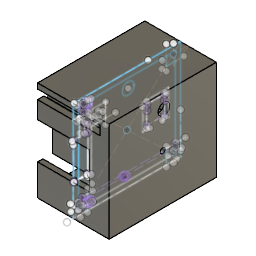
Light and Temp sensor v1 (Autodesk Fusion 360 design; units mm, degrees)
Autodesk Fusion 360 part; units mm, degrees
sketch "DHT22" plane through (0, 0, 0) normal (0, 0, 1) x (1, 0, 0)
  line L0 (7.5, -10) -> (-7.5, -10)
  line L1 (-7.5, -10) -> (-7.5, 10)
  line L2 (-7.5, 10) -> (7.5, 10)
  line L3 (7.5, 10) -> (7.5, -10)
  line L4 (7.5, -10) -> (-7.5, 10) construction
  line L5 (-7.5, -10) -> (7.5, 10) construction
  line L6 (-16.1042, 15) -> (19.3546, 15) construction
  line L7 (7.5, 10) -> (4.6132, 15)
  line L8 (0, -2.0118) -> (0, 2.0118) construction
  line L9 (-3.2444, 0) -> (3.2444, 0) construction
  line L10 (-7.5, 10) -> (-4.6132, 15)
  line L11 (-4.6132, 15) -> (4.6132, 15)
  line L12 (-8.5762, 12.5) -> (8.9313, 12.5) construction
  line L13 (0, 15.9476) -> (0, 9.0438) construction
  circle A0 centre (0, 12.4957) radius 1.4
  line L14 (-5.5335, -10) -> (-5.5335, -18)
  line L15 (-5.0335, -10) -> (-5.0335, -18)
  line L16 (-5.5335, -18) -> (-5.0335, -18)
  line L17 (-1.7002, -10) -> (-1.7002, -18)
  line L18 (-2.2002, -18) -> (-1.7002, -18)
  line L19 (-2.2002, -10) -> (-2.2002, -18)
  line L20 (1.6331, -10) -> (1.6331, -18)
  line L21 (1.1331, -18) -> (1.6331, -18)
  line L22 (1.1331, -10) -> (1.1331, -18)
  line L23 (4.9665, -10) -> (4.9665, -18)
  line L24 (4.4665, -18) -> (4.9665, -18)
  line L25 (4.4665, -10) -> (4.4665, -18)
  dimension "d1" = 15
  dimension "d2" = 20
  dimension "d3" = 15
  dimension "d4" = 60
  dimension "d5" = 2.8
  dimension "d6" = 8
  dimension "d7" = 0.5
  dimension "d10" = 10
  dimension "d11" = 0
  constraint horizontal L0
  constraint perpendicular L0 L1
  constraint parallel L0 L2
  constraint parallel L1 L3
  constraint coincident L4 origin
  constraint coincident L5 origin
  constraint perpendicular L1 L6
  constraint coincident L6 L7.end
  constraint vertical L8
  constraint perpendicular L8 L9
  constraint midpoint origin L8
  constraint midpoint origin L9
  constraint symmetric L2.end L8 L1.end
  constraint symmetric L7.end L8 L10.end
  constraint horizontal L12
  constraint perpendicular L12 L13
  constraint symmetric L2.end L1.end L13
  constraint midpoint L13 A0.centre
  constraint coincident L0 L14.start
  constraint perpendicular L0 L14
  constraint coincident L0 L15.start
  constraint perpendicular L0 L15
  constraint equal L14 L15
  measures "d1" distance of L1.end L2.end
  measures "d2" distance of L0.end L1.end
  measures "d3" distance of origin L6
  measures "d4" angle of L6 L7
  measures "d5" diameter of A0
  measures "d6" distance of L0 L14.end
  measures "d7" distance of L14 L15
extrude "Extrude1" add sketch "DHT22" along normal blind 7.7 contours L0 L1 L2 L3 makes body 1 in component "DHT22"
extrude "Extrude2" add sketch "DHT22" along normal blind 1.5 contours L2 L7 L10 L11 bodies 1 in component "DHT22"
extrude "Extrude3" add sketch "DHT22" along normal blind 4.1 and the other way blind -3.6 contours L0 L23 L24 L25 | L0 L20 L21 L22 | L0 L14 L15 L16 | L0 L17 L18 L19 bodies 1 in component "DHT22"
sketch "Light sensor" plane through (0, 0, 0) normal (0, 0, 1) x (1, 0, 0)
  line L0 (-2.4, 4.9216) -> (-2.4, -4.8279) construction
  line L1 (2.4, 4.9216) -> (2.4, -4.8279) construction
  line L2 (-3.4686, 2.05) -> (2.8124, 2.05) construction
  line L3 (-3.4686, -2.05) -> (1.4, -2.05) construction
  line L4 (0, -1.3974) -> (0, 1.3974) construction
  line L5 (1.6915, 0) -> (-1.6915, 0) construction
  line L6 (-1.4, 2.05) -> (1.4, 2.05)
  line L7 (2.4, 1.05) -> (2.4, -1.05)
  line L8 (2.4, -2.05) -> (-1.4, -2.05)
  line L9 (-2.4, -1.05) -> (-2.4, 1.05)
  arc A0 (-1.4, 2.05) -> (-2.4, 1.05) centre (-1.4, 1.05) ccw
  arc A1 (2.4, 1.05) -> (1.4, 2.05) centre (1.4, 1.05) ccw
  arc A2 (-2.4, -1.05) -> (-1.4, -2.05) centre (-1.4, -1.05) ccw
  arc A3 (1.4, -2.05) -> (2.4, -1.05) centre (1.4, -1.05) ccw
  circle A4 centre (-1.9, 0) radius 0.15
  circle A5 centre (1.9, 0) radius 0.15
  dimension "d20" = 4.8
  dimension "d21" = 4.1
  dimension "d22" = 1
  dimension "d23" = 1
  dimension "d24" = 1
  dimension "d25" = 1
  dimension "d26" = 0.3
  dimension "d27" = 0.5
  constraint vertical L0
  constraint parallel L0 L1
  constraint perpendicular L0 L2
  constraint perpendicular L0 L3
  constraint perpendicular L3 L4
  constraint perpendicular L1 L5
  constraint midpoint origin L5
  constraint midpoint origin L4
  constraint horizontal L6
  constraint vertical L7
  constraint horizontal L8
  constraint vertical L9
  constraint coincident L1 L8.start
  constraint coincident L3 L8.start
  constraint tangent L6 A0
  constraint tangent L9 A0
  constraint tangent L6 A1
  constraint tangent L7 A1
  constraint tangent L8 A2
  constraint tangent L9 A2
  constraint coincident L8.start L7
  constraint tangent L7 A3
  constraint tangent L3 A3
  constraint symmetric L4 A4 A5
  measures "d20" distance of L0 L1
  measures "d21" distance of L2 L3
  measures "d22" radius of A0
  measures "d23" radius of A1
  measures "d24" radius of A2
  measures "d25" radius of A3
  measures "d26" diameter of A4
  measures "d27" distance of L0 A4.centre
extrude "Extrude1'" add sketch "Light sensor" along normal blind 2.3 separate body contours L6 L7 L8 L9 A0 A1 A2 A3 | A4 | A5 makes body 2 in component "Light sensor"
extrude "Extrude2'" add sketch "Light sensor" against normal blind 30 contours A4 | A5 bodies 2 in component "Light sensor"
sketch "ESP32 Wroom-32" plane through (0, 0, 0) normal (0, 0, 1) x (1, 0, 0)
  line L0 (14.1, -44.2458) -> (14.1, 38.8499) construction
  line L1 (-14.1, -44.2458) -> (-14.1, 38.8499) construction
  line L2 (0, -14.9734) -> (0, 14.9734) construction
  line L3 (8.9037, 0) -> (-8.9037, 0) construction
  line L4 (24.487, -25.95) -> (-46.8728, -25.95) construction
  line L5 (24.487, 25.95) -> (-46.8728, 25.95) construction
  line L6 (14.1, -25.95) -> (-14.1, -25.95)
  line L7 (-14.1, -25.95) -> (-14.1, 25.95)
  line L8 (-14.1, 25.95) -> (14.1, 25.95)
  line L9 (14.1, 25.95) -> (14.1, -25.95)
  circle A0 centre (11.3, -23.15) radius 1.6
  circle A1 centre (-11.3, -23.15) radius 1.6
  circle A2 centre (11.3, 23.15) radius 1.6
  circle A3 centre (-11.3, 23.15) radius 1.6
  line L10 (4.4, 20.65) -> (-4.4, 20.65)
  line L11 (-4.4, 20.65) -> (-4.4, 28.05)
  line L12 (-4.4, 28.05) -> (4.4, 28.05)
  line L13 (4.4, 28.05) -> (4.4, 20.65)
  line L14 (8.9, 20.35) -> (6.3, 20.35)
  line L15 (6.3, 20.35) -> (6.3, 24.25)
  line L16 (6.3, 24.25) -> (8.9, 24.25)
  line L17 (8.9, 24.25) -> (8.9, 20.35)
  line L18 (7.6, 22.1367) -> (7.6, 22.6573) construction
  line L19 (8.0941, 22.3) -> (7.6065, 22.3) construction
  circle A4 centre (7.6, 22.3) radius 0.8
  line L20 (15.8445, 24.25) -> (-17.3175, 24.25) construction
  line L21 (-8.9, 24.25) -> (-8.9, 20.35)
  line L22 (-8.9, 20.35) -> (-6.3, 20.35)
  line L23 (-6.3, 20.35) -> (-6.3, 24.25)
  line L24 (-6.3, 24.25) -> (-8.9, 24.25)
  circle A5 centre (-7.6, 22.3) radius 0.8
  line L25 (-3.8, 2.05) -> (-5.8, 2.05)
  line L26 (-5.8, 2.05) -> (-5.8, 3.05)
  line L27 (-5.8, 3.05) -> (-3.8, 3.05)
  line L28 (-3.8, 3.05) -> (-3.8, 2.05)
  line L29 (2.9, 2.05) -> (0.9, 2.05)
  line L30 (0.9, 2.05) -> (0.9, 3.05)
  line L31 (0.9, 3.05) -> (2.9, 3.05)
  line L32 (2.9, 3.05) -> (2.9, 2.05)
  line L33 (13.9, -20.75) -> (11.4, -20.75)
  line L34 (11.4, -20.75) -> (11.4, 17.15)
  line L35 (11.4, 17.15) -> (13.9, 17.15)
  line L36 (13.9, 17.15) -> (13.9, -20.75)
  line L37 (-11.4, -20.75) -> (-11.4, 17.15)
  line L38 (-13.9, -20.75) -> (-11.4, -20.75)
  line L39 (-13.9, 17.15) -> (-13.9, -20.75)
  line L40 (-11.4, 17.15) -> (-13.9, 17.15)
  dimension "d34" = 51.9
  dimension "d35" = 28.2
  dimension "d36" = 3.2
  dimension "d37" = 2.8
  dimension "d38" = 2.8
  dimension "d39" = 8.8
  dimension "d40" = 7.4
  dimension "d41" = 2.1
  dimension "d42" = 2.6
  dimension "d43" = 3.9
  dimension "d44" = 1.6
  dimension "d45" = 1.7
  dimension "d46" = 1.9
  dimension "d47" = 2
  dimension "d48" = 1
  dimension "d49" = 8.3
  dimension "d50" = 22.9
  dimension "d51" = 2
  dimension "d52" = 1
  dimension "d53" = 4.7
  dimension "d54" = 2.5
  dimension "d55" = 37.9
  dimension "d56" = 8.8
  dimension "d57" = 0.2
  constraint vertical L0
  constraint parallel L0 L1
  constraint parallel L1 L2
  constraint perpendicular L2 L4
  constraint perpendicular L0 L5
  constraint symmetric L0 L1 L2
  constraint midpoint origin L2
  constraint midpoint origin L3
  constraint symmetric L3 L4 L5
  constraint horizontal L6
  constraint vertical L7
  constraint horizontal L8
  constraint vertical L9
  constraint coincident L5 L7.end
  constraint coincident L1 L7.end
  constraint coincident L4 L6.start
  constraint coincident L0 L6.start
  constraint symmetric L2 A0 A1
  constraint symmetric L3 A0 A2
  constraint symmetric L3 A1 A3
  constraint horizontal L10
  constraint vertical L11
  constraint horizontal L12
  constraint vertical L13
  constraint symmetric L2 L11 L13
  constraint horizontal L14
  constraint vertical L15
  constraint horizontal L16
  constraint vertical L17
  constraint vertical L18
  constraint perpendicular L18 L19
  constraint symmetric L14 L16 L19
  constraint symmetric L15 L17 L18
  constraint coincident L18 A4.centre
  constraint coincident L19 A4.centre
  constraint perpendicular L9 L20
  constraint collinear L16 L20
  constraint symmetric L2 L14.start L21.end
  constraint symmetric L2 L14.end L22.end
  constraint symmetric L2 L15.end L23.end
  constraint symmetric L2 L16.end L21.start
  constraint symmetric L2 A4 A5
  constraint horizontal L25
  constraint vertical L26
  constraint horizontal L27
  constraint vertical L28
  constraint horizontal L29
  constraint vertical L30
  constraint horizontal L31
  constraint vertical L32
  constraint collinear L27 L31
  constraint horizontal L33
  constraint vertical L34
  constraint horizontal L35
  constraint vertical L36
  constraint symmetric L2 L33.start L38.start
  constraint symmetric L2 L33.end L37.start
  constraint symmetric L2 L34.end L37.end
  constraint symmetric L2 L35.end L39.start
  measures "d34" distance of L4 L5
  measures "d35" distance of L0 L1
  measures "d36" diameter of A0
  measures "d37" distance of L6 A0.centre
  measures "d38" distance of L0 A0.centre
  measures "d39" distance of L10.start L10.end
  measures "d40" distance of L10.start L12.end
  measures "d41" distance of L8 L12
  measures "d42" distance of L14.start L14.end
  measures "d43" distance of L14.start L16.end
  measures "d44" diameter of A4
  measures "d45" distance of L5 L20
  measures "d46" distance of L13 L15
  measures "d47" distance of L25.start L25.end
  measures "d48" distance of L25.start L27.end
  measures "d49" distance of L7 L26
  measures "d50" distance of L8 L27
  measures "d51" distance of L29.start L29.end
  measures "d52" distance of L29.start L31.end
  measures "d53" distance of L28 L30
  measures "d54" distance of L33.start L33.end
  measures "d55" distance of L33.start L35.end
  measures "d56" distance of L8 L35
  measures "d57" distance of L0 L36
extrude "Extrude1''" add sketch "ESP32 Wroom-32" along normal blind 1.5 separate body contours L6 L7 L8 L9 L10 L11 L13 | L8 L10 L11 L13 | L14 L15 L16 L17 | A4 | L21 L22 L23 L24 | A5 | L25 L26 L27 L28 | L29 L30 L31 L32 | L33 L34 L35 L36 | L37 L38 L39 L40 makes body 3 in component "ESP32 Wroom-32"
extrude "Extrude2''" add sketch "ESP32 Wroom-32" along normal blind 4.7 and the other way blind -1.5 contours L8 L10 L11 L13 | L8 L11 L12 L13 bodies 3 in component "ESP32 Wroom-32"
extrude "Extrude3'" add sketch "ESP32 Wroom-32" along normal blind 3.5 and the other way blind -1.5 contours L14 L15 L16 L17 | A4 | L21 L22 L23 L24 | A5 bodies 3 in component "ESP32 Wroom-32"
extrude "Extrude4" add sketch "ESP32 Wroom-32" along normal blind 4.2 and the other way blind -1.5 contours A4 | A5 bodies 3 in component "ESP32 Wroom-32"
extrude "Extrude5" add sketch "ESP32 Wroom-32" along normal blind 2 and the other way blind -1.5 contours L25 L26 L27 L28 | L29 L30 L31 L32 bodies 3 in component "ESP32 Wroom-32"
extrude "Extrude6" add sketch "ESP32 Wroom-32" against normal blind 8.3 contours L33 L34 L35 L36 | L37 L38 L39 L40 bodies 3 in component "ESP32 Wroom-32"
sketch "Screw terminal" plane through (0, 0, 0) normal (0, 0, 1) x (1, 0, 0)
  line L0 (4.9, -4.95) -> (-4.9, -4.95)
  line L1 (-4.9, -4.95) -> (-4.9, 4.95)
  line L2 (-4.9, 4.95) -> (4.9, 4.95)
  line L3 (4.9, 4.95) -> (4.9, -4.95)
  line L4 (0, 1.4194) -> (0, -1.4194) construction
  line L5 (-1.4426, 0) -> (1.4426, 0) construction
  line L6 (4.6, -0.85) -> (0.4, -0.85)
  line L7 (0.4, -0.85) -> (0.4, 4.55)
  line L8 (0.4, 4.55) -> (4.6, 4.55)
  line L9 (4.6, 4.55) -> (4.6, -0.85)
  line L10 (-4.6, 4.55) -> (-4.6, -0.85)
  line L11 (-4.6, -0.85) -> (-0.4, -0.85)
  line L12 (-0.4, -0.85) -> (-0.4, 4.55)
  line L13 (-0.4, 4.55) -> (-4.6, 4.55)
  line L14 (2.65, 4.95) -> (2.35, 4.95)
  line L15 (2.35, 4.95) -> (2.35, 8.45)
  line L16 (2.35, 8.45) -> (2.65, 8.45)
  line L17 (2.65, 8.45) -> (2.65, 4.95)
  line L18 (2.5, 7.4653) -> (2.5, 5.947) construction
  line L19 (-2.35, 4.95) -> (-2.35, 8.45)
  line L20 (-2.65, 4.95) -> (-2.35, 4.95)
  line L21 (-2.65, 8.45) -> (-2.65, 4.95)
  line L22 (-2.35, 8.45) -> (-2.65, 8.45)
  dimension "d78" = 9.8
  dimension "d79" = 9.9
  dimension "d80" = 4.2
  dimension "d81" = 5.4
  dimension "d82" = 4.1
  dimension "d83" = 0.3
  dimension "d84" = 0.3
  dimension "d85" = 3.5
  constraint horizontal L0
  constraint vertical L1
  constraint horizontal L2
  constraint vertical L3
  constraint parallel L1 L4
  constraint perpendicular L4 L5
  constraint midpoint origin L5
  constraint midpoint origin L4
  constraint symmetric L0 L2 L5
  constraint symmetric L1 L3 L4
  constraint horizontal L6
  constraint vertical L7
  constraint horizontal L8
  constraint vertical L9
  constraint symmetric L4 L6.start L10.end
  constraint symmetric L4 L6.end L11.end
  constraint symmetric L4 L7.end L12.end
  constraint symmetric L4 L8.end L10.start
  constraint horizontal L14
  constraint vertical L15
  constraint horizontal L16
  constraint vertical L17
  constraint coincident L2 L14.start
  constraint perpendicular L16 L18
  constraint symmetric L15 L17 L18
  constraint symmetric L7 L9 L18
  constraint symmetric L4 L14.start L20.start
  constraint symmetric L4 L14.end L19.start
  constraint symmetric L4 L15.end L19.end
  constraint symmetric L4 L16.end L21.start
  measures "d78" distance of L0.start L0.end
  measures "d79" distance of L0.start L2.end
  measures "d80" distance of L6.start L6.end
  measures "d81" distance of L6.start L8.end
  measures "d82" distance of L0 L6
  measures "d83" distance of L3 L9
  measures "d84" distance of L14.start L14.end
  measures "d85" distance of L14.start L16.end
extrude "Extrude1'''" add sketch "Screw terminal" along normal blind 7.7 separate body contours L0 L1 L2 L3 L14 L20 | L6 L7 L8 L9 | L10 L11 L12 L13 makes body 4 in component "Screw terminal"
extrude "Extrude2'''" cut sketch "Screw terminal" along normal blind 8 and the other way blind -5 contours L6 L7 L8 L9 | L10 L11 L12 L13 bodies 4 in component "Screw terminal"
extrude "Extrude3''" add sketch "Screw terminal" along normal blind 4.15 and the other way blind -3.85 contours L2 L14 L15 L16 L17 | L2 L19 L20 L21 L22 bodies 4 in component "Screw terminal"
sketch "Sketch1" plane through (0, 0, 0) normal (1, 0, 0) x (0, 1, 0) in component "Screw terminal"
  line L0 (4.95, 0) -> (-4.95, 0)
  line L1 (-4.95, 0) -> (-4.95, 7.7)
  line L2 (-4.95, 7.7) -> (4.95, 7.7)
  line L3 (4.95, 7.7) -> (4.95, 0)
  line L4 (-2.05, 9.7062) -> (-2.05, -0.1924) construction
  line L5 (-6.0619, 6.7) -> (-1.5708, 6.7) construction
  line L6 (-6.0619, 1.7) -> (-1.5708, 1.7) construction
  line L7 (-2.05, 7.7) -> (-4.95, 6.7)
  line L8 (-2.05, 0) -> (-4.95, 1.7)
  line L9 (-2.05, 0) -> (-4.95, 0)
  line L10 (-4.95, 0) -> (-4.95, 1.7)
  line L11 (-4.95, 6.7) -> (-4.95, 7.7)
  line L12 (-4.95, 7.7) -> (-2.05, 7.7)
  dimension "d96" = 7
  dimension "d97" = 5
  dimension "d98" = 1
  constraint perpendicular L0 L4
  constraint perpendicular L4 L5
  constraint perpendicular L4 L6
  constraint coincident L4 L7.start
  constraint coincident L2 L7.start
  constraint coincident L1 L7.end
  constraint coincident L5 L7.end
  constraint coincident L0 L8.start
  constraint coincident L4 L8.start
  constraint coincident L1 L8.end
  constraint coincident L6 L8.end
  constraint coincident L0.end L1.start
  constraint coincident L1.end L2.start
  measures "d96" distance of L3 L4
  measures "d97" distance of L5 L6
  measures "d98" distance of L2 L5
extrude "Extrude4'" cut sketch "Sketch1" along normal mid plane 10 contours L0 L1 L8 L9 L10 | L1 L2 L7 L11 L12 bodies 4 in component "Screw terminal"
sketch "Sketch2" plane through (0, -4.95, 0) normal (0, -1, 0) x (1, 0, 0) in component "Screw terminal"
  line L0 (4.9, 6.7) -> (-4.9, 6.7)
  line L1 (-4.9, 6.7) -> (-4.9, 1.7)
  line L2 (-4.9, 1.7) -> (4.9, 1.7)
  line L3 (4.9, 1.7) -> (4.9, 6.7)
  line L4 (-5.6068, 4.2) -> (5.7003, 4.2) construction
  line L5 (-2.4483, -0.8504) -> (-2.4483, 8.9242) construction
  line L6 (0.0034, -0.7898) -> (0.0034, 0.468) construction
  line L7 (-4.9, 1.7) -> (-4.9, 6.7) construction
  line L8 (4.9, 1.7) -> (4.9, 6.7) construction
  line L9 (-4.9, 1.7) -> (4.9, 1.7) construction
  line L10 (4.9, 6.7) -> (-4.9, 6.7) construction
  circle A0 centre (-2.4483, 4.2) radius 1.75
  circle A1 centre (2.4551, 4.2) radius 1.75
  dimension "d101" = 3.5
  constraint perpendicular L3 L4
  constraint perpendicular L2 L5
  constraint perpendicular L2 L6
  constraint symmetric L0 L4 L9
  constraint coincident L5 A0.centre
  constraint coincident L4 A0.centre
  constraint symmetric L6 A0 A1
  measures "d101" diameter of A0
extrude "Extrude5'" cut sketch "Sketch2" against normal blind 6.5 contours A0 | A1 bodies 4 in component "Screw terminal"
sketch "Box side view" plane through (0, 0, 0) normal (1, 0, 0) x (0, 1, 0)
  line L0 (26.8145, -7.7) -> (-34.5766, -7.7) construction
  line L1 (28.95, -4.6875) -> (28.95, 15.0705) construction
  line L2 (-31.05, -1.5625) -> (-31.05, 27.8729) construction
  line L3 (-20.6653, 4.0827) -> (-20.6653, 36.4415) construction
  line L4 (-27.5, 32.006) -> (-27.5, 37.8528) construction
  line L5 (-30.6451, 48.05) -> (10.7863, 48.05) construction
  line L6 (-28.05, -4.7) -> (-20.65, -4.7) construction
  line L7 (-25.95, -1.5) -> (25.95, -1.5) construction
  line L8 (25.95, 0) -> (-25.95, 0) construction
  line L9 (-30.7, 30) -> (-30.7, 10) construction
  line L10 (-23, 10) -> (-23, 30) construction
  line L11 (-23, 30) -> (-23, 35) construction
  line L12 (-24.5, 35) -> (-24.5, 30) construction
  line L13 (-23, 10) -> (-30.7, 10) construction
  line L14 (10.1, 17.05) -> (10.1, 24.05) construction
  line L15 (19.9, 17.05) -> (10.1, 17.05) construction
  line L16 (19.9, 24.05) -> (19.9, 17.05) construction
  line L17 (25.95, 0) -> (25.95, -1.5) construction
  line L18 (-25.95, 0) -> (-25.95, -1.5) construction
  line L19 (-28.05, -1.5) -> (-28.05, -4.7) construction
  line L20 (-3.05, -2) -> (-2.05, -2) construction
  line L21 (-2.05, -1.5) -> (-2.05, -2) construction
  line L22 (-3.05, -1.5) -> (-3.05, -2) construction
  line L23 (-23.1, -4.2) -> (-21.5, -4.2) construction
  line L24 (-21.5, -3.5) -> (-23.1, -3.5) construction
  line L25 (19.9, 24.05) -> (19.9, 26.95) construction
  line L26 (19.9, 26.95) -> (10.1, 26.95) construction
  line L27 (10.1, 26.95) -> (10.1, 24.05) construction
  line L28 (-23, 35) -> (-24.5, 35) construction
  line L29 (-24.5, 30) -> (-30.7, 30) construction
  line L30 (-23, 40.95) -> (-25.3, 40.95) construction
  line L31 (-23, 41.95) -> (-23, 44.05) construction
  line L32 (-25.3, 44.05) -> (-25.3, 41.95) construction
  line L33 (-23, 45.05) -> (-25.3, 45.05) construction
  line L34 (-31.05, -7.7) -> (-31.05, 48.05)
  line L35 (-31.05, 48.05) -> (28.95, 48.05)
  line L36 (-31.05, -7.7) -> (28.95, -7.7)
  line L37 (28.95, -7.7) -> (28.95, 48.05)
  line L38 (25.95, -4.7) -> (25.95, 45.05)
  line L39 (-28.05, 45.05) -> (25.95, 45.05)
  line L40 (-28.05, -4.7) -> (-28.05, 45.05)
  line L41 (-28.05, -4.7) -> (25.95, -4.7)
  line L42 (-28.9766, 37.95) -> (-22.6639, 37.95) construction
  line L43 (-21, 45.4212) -> (-21, 39.95) construction
  line L44 (-23, 41.95) -> (-23, 40.95) construction
  line L45 (-29.0303, 46.05) -> (-24.1853, 46.05) construction
  line L46 (-27.5, 46.5514) -> (-27.5, 39.1534) construction
  line L47 (-25.3, 35.2) -> (-22.8, 35.2) construction
  line L48 (-24.7, 35.9637) -> (-24.7, 30.5464) construction
  line L49 (-31.7083, 30.2) -> (-24.7, 30.2) construction
  line L50 (-22.8, 34.0029) -> (-22.8, 8.4261) construction
  line L51 (-30.7, 9.8) -> (-23.4352, 9.8) construction
  line L52 (-22.8, 45.7046) -> (-22.8, 39.81) construction
  line L53 (-22.8, 42.4599) -> (-21, 42.4599)
  line L54 (-22.8, 42.4599) -> (-22.8, 39.95)
  line L55 (-21, 42.4599) -> (-21, 39.95)
  line L56 (-22.8, 43.7599) -> (-21, 43.7599)
  line L57 (-22.8, 43.7599) -> (-22.8, 45.05)
  line L58 (-21, 43.7599) -> (-21, 45.05)
  line L59 (-31.05, 39.95) -> (-25.3, 39.95) construction
  line L60 (-25.3, 39.95) -> (-21, 39.95)
  line L61 (-25.3, 40.95) -> (-25.3, 37.95) construction
  line L62 (-25.3, 37.95) -> (-25.3, 39.95)
  line L63 (-25.3, 37.95) -> (-25.3, 35.2)
  line L64 (-25.3, 35.2) -> (-22.8, 35.2)
  line L65 (-21, 39.95) -> (-21, 8.6323)
  line L66 (-22.8, 9.8) -> (-22.8, 35.2)
  line L67 (-27.5, 39.95) -> (-28.05, 39.95)
  line L68 (-27.5, 39.95) -> (-27.5, 30.2)
  line L69 (-27.5, 30.2) -> (-24.7, 30.2)
  line L70 (-24.7, 35.2) -> (-24.7, 30.2)
  line L71 (-27.5, 45.05) -> (-27.5, 46.05)
  line L72 (-27.5, 46.05) -> (-25.3106, 46.05)
  line L73 (-25.3, 45.05) -> (-25.3106, 46.05)
  line L74 (-28.05, 39.95) -> (-31.05, 39.95)
  line L75 (-28.05, 45.05) -> (-31.05, 45.05)
  line L76 (-25.3, 37.95) -> (-28.05, 37.95)
  line L77 (-27.5, 30.2) -> (-28.05, 30.2)
  line L78 (-25.8444, 9.8) -> (-21, 9.8)
  line L79 (-31.05, 9.8) -> (-28.05, 9.8)
  line L80 (-28.05, 30.2) -> (-31.05, 30.2)
  circle A0 centre (-0.3533, 40.05) radius 3.25
  line L81 (9.9, 15.3744) -> (9.9, 28.8283) construction
  line L82 (20.1, 16.0643) -> (20.1, 28.009) construction
  line L83 (20.887, 27.15) -> (7.4762, 27.15) construction
  line L84 (19.1, 16.85) -> (10.9, 16.85) construction
  line L85 (20.1, 27.15) -> (9.9, 27.15)
  line L86 (11.6455, 16.85) -> (9.9, 16.85)
  line L87 (9.9, 27.15) -> (9.9, 16.85)
  line L88 (18.6483, 16.85) -> (20.1, 16.85)
  line L89 (20.1, 16.85) -> (20.1, 27.15)
  line L90 (18.6483, 14.85) -> (22.1, 14.85)
  line L91 (22.1, 14.85) -> (22.1, 29.15)
  line L92 (22.1, 29.15) -> (7.9, 29.15)
  line L93 (7.9, 29.15) -> (7.9, 14.85)
  line L94 (11.6455, 14.85) -> (7.9, 14.85)
  line L95 (19.1, 16.85) -> (19.1, 14.85)
  line L96 (10.9, 16.85) -> (10.9, 14.85)
  line L97 (26.15, 0.885) -> (26.15, -1.9462) construction
  line L98 (-20.3044, -4.9) -> (-28.4281, -4.9) construction
  line L99 (-28.25, -0.9057) -> (-28.25, -5.03) construction
  line L100 (25.95, 0) -> (26.15, 0)
  line L101 (26.15, 0) -> (26.15, -1.5)
  line L102 (25.95, -1.5) -> (26.15, -1.5)
  line L103 (-20.65, -4.7) -> (-20.65, -4.9)
  line L104 (-28.05, -1.5) -> (-28.25, -1.5)
  line L105 (-28.25, -1.5) -> (-28.25, -4.9)
  line L106 (-28.25, -4.9) -> (-20.65, -4.9)
  line L107 (-25.8444, 9.8) -> (-28.05, 9.8)
  line L108 (-24.7, 30.2) -> (-21, 30.2)
  line L109 (-25.3, 39.95) -> (-25.3, 45.05)
  line L110 (-22.8, 42.4599) -> (-22.8, 43.7599)
  line L111 (-21, 42.4599) -> (-21, 43.7599)
  line L112 (30.761, 40.05) -> (18.4258, 40.05) construction
  line L113 (20.95, 50.8354) -> (20.95, 37.6777) construction
  line L114 (25.95, 40.05) -> (20.95, 40.05)
  line L115 (20.95, 40.05) -> (20.95, 45.05)
  line L116 (24.95, 49.1649) -> (24.95, 38.3029) construction
  line L117 (24.95, 38.3029) -> (33.6431, 44.05) construction
  line L118 (33.6431, 44.05) -> (18.6993, 44.05) construction
  circle A1 centre (24.95, 44.05) radius 1.4
  line L119 (20.95, -8.7658) -> (20.95, 1.4637) construction
  line L120 (31.6256, 0.3) -> (20.9786, 0.3) construction
  line L121 (29.6274, -3.7) -> (21.8136, -3.7) construction
  line L122 (24.95, -8.6792) -> (24.95, -2.6614) construction
  line L123 (20.9786, 0.3) -> (20.95, -7.7)
  line L124 (20.9786, 0.3) -> (28.95, 0.3)
  circle A2 centre (24.95, -3.7) radius 1.4
  line L125 (-23.05, -8.6297) -> (-23.05, 2.7565) construction
  line L126 (-32.711, 0.3) -> (-20.1818, 0.3) construction
  line L127 (-27.05, -9.0254) -> (-27.05, -2.9362) construction
  line L128 (-32.4059, -3.7) -> (-25.9641, -3.7) construction
  line L129 (-23.05, -7.7) -> (-23.05, 0.3)
  line L130 (-23.05, 0.3) -> (-31.05, 0.3)
  circle A3 centre (-27.05, -3.7) radius 1.4
  line L131 (-13, 28.7001) -> (-13, 39.8567) construction
  line L132 (-7.486, 31.95) -> (-18.7673, 31.95) construction
  line L133 (-13, 31.95) -> (-21, 31.95)
  line L134 (-21, 31.95) -> (-21, 39.95)
  line L135 (-21, 39.95) -> (-13, 39.95)
  line L136 (-13, 39.95) -> (-13, 31.95)
  line L137 (-17, 37.5203) -> (-17, 34.1536) construction
  line L138 (-14.5483, 35.95) -> (-18.8052, 35.95) construction
  circle A4 centre (-17, 35.95) radius 1.4
  line L139 (-31.05, 48.05) -> (28.95, -7.7) construction
  line L140 (28.95, 48.05) -> (-31.05, -7.7) construction
  circle A5 centre (-1.05, 20.175) radius 1.4
  dimension "d104" = 3
  dimension "d105" = 3
  dimension "d106" = 3
  dimension "d107" = 3
  dimension "d108" = 3
  dimension "d109" = 3
  dimension "d116" = 3
  dimension "d117" = 2
  dimension "d118" = 1
  dimension "d119" = 2.2
  dimension "d120" = 0.2
  dimension "d121" = 0.2
  dimension "d122" = 0.2
  dimension "d123" = 0.2
  dimension "d124" = 0.2
  dimension "d125" = 0.2
  dimension "d127" = 1.3
  dimension "d128" = 1
  dimension "d129" = 6.5
  dimension "d130" = 5
  dimension "d131" = 0.2
  dimension "d132" = 0.2
  dimension "d133" = 0.2
  dimension "d134" = 0.2
  dimension "d135" = 2
  dimension "d136" = 3
  dimension "d137" = 3
  dimension "d138" = 0.2
  dimension "d139" = 0.2
  dimension "d140" = 0.2
  dimension "d187" = 8
  dimension "d188" = 8
  dimension "d189" = 2.8
  dimension "d190" = 8
  dimension "d191" = 8
  dimension "d192" = 4
  dimension "d193" = 4
  dimension "d194" = 2.8
  dimension "d195" = 8
  dimension "d196" = 8
  dimension "d197" = 4
  dimension "d198" = 4
  dimension "d199" = 2.8
  dimension "d200" = 8
  dimension "d201" = 8
  dimension "d202" = 2.8
  dimension "d221" = 2.8
  constraint horizontal L0
  constraint perpendicular L0 L1
  constraint perpendicular L0 L2
  constraint perpendicular L0 L3
  constraint parallel L3 L4
  constraint perpendicular L3 L5
  constraint coincident L0 L34.start
  constraint perpendicular L13 L34
  constraint perpendicular L3 L35
  constraint perpendicular L34 L36
  constraint perpendicular L35 L37
  constraint horizontal L42
  constraint parallel L9 L43
  constraint perpendicular L40 L45
  constraint perpendicular L45 L46
  constraint perpendicular L3 L47
  constraint perpendicular L47 L48
  constraint perpendicular L40 L49
  constraint perpendicular L13 L50
  constraint perpendicular L40 L51
  constraint perpendicular L30 L52
  constraint coincident L52 L53.start
  constraint coincident L43 L53.end
  constraint perpendicular L43 L53
  constraint coincident L43 L55.end
  constraint coincident L43 L56.end
  constraint perpendicular L43 L56
  constraint coincident L52 L57.end
  constraint coincident L39 L57.end
  constraint perpendicular L39 L57
  constraint coincident L43 L58.end
  constraint coincident L39 L58.end
  constraint perpendicular L52 L59
  constraint perpendicular L43 L60
  constraint coincident L54.end L60
  constraint coincident L43.end L55.end
  constraint coincident L30.end L61.start
  constraint coincident L42 L61.end
  constraint perpendicular L42 L61
  constraint coincident L61 L59.end
  constraint coincident L59.end L61
  constraint coincident L59.end L60.start
  constraint perpendicular L42 L63
  constraint perpendicular L3 L64
  constraint perpendicular L60 L65
  constraint coincident L50 L66.start
  constraint coincident L50 L47.end
  constraint coincident L64 L47.end
  constraint coincident L47.end L64.end
  constraint coincident L34 L59.start
  constraint coincident L46 L67.start
  constraint coincident L59 L67.start
  constraint coincident L59 L67.end
  constraint coincident L40 L67.end
  constraint coincident L49 L68.end
  constraint perpendicular L49 L68
  constraint coincident L49 L69.end
  constraint coincident L64 L70.start
  constraint perpendicular L64 L70
  constraint collinear L48 L70
  constraint coincident L49.end L69.end
  constraint coincident L46 L71.start
  constraint coincident L39 L71.start
  constraint coincident L45 L71.end
  constraint coincident L46 L71.end
  constraint coincident L45 L72.end
  constraint coincident L33.end L73.start
  constraint coincident L34 L75.end
  constraint perpendicular L34 L75
  constraint coincident L42 L76.end
  constraint coincident L40 L76.end
  constraint coincident L49 L77.end
  constraint coincident L40 L77.end
  constraint coincident L51 L78.start
  constraint coincident L65 L78.end
  constraint perpendicular L65 L78
  constraint coincident L51 L79.start
  constraint coincident L51 L79.end
  constraint coincident L40 L79.end
  constraint coincident L34 L79.start
  constraint coincident L66.start L78
  constraint coincident L49 L80.end
  constraint coincident L34 L80.end
  constraint coincident L47.start L63.end
  constraint parallel L4 L81
  constraint vertical L82
  constraint horizontal L83
  constraint perpendicular L82 L84
  constraint coincident L82 L85.start
  constraint coincident L83 L85.start
  constraint coincident L81 L85.end
  constraint coincident L83 L85.end
  constraint coincident L84 L86.start
  constraint coincident L81 L86.end
  constraint perpendicular L81 L86
  constraint coincident L84 L88.start
  constraint coincident L82 L88.end
  constraint perpendicular L82 L88
  constraint coincident L90 L95.end
  constraint perpendicular L90 L95
  constraint coincident L94 L96.end
  constraint perpendicular L94 L96
  constraint perpendicular L8 L97
  constraint perpendicular L34 L98
  constraint perpendicular L0 L99
  constraint coincident L8.start L17.start
  constraint coincident L97 L100.end
  constraint perpendicular L97 L100
  constraint coincident L97 L101.end
  constraint coincident L7.end L17.end
  constraint perpendicular L97 L102
  constraint coincident L101.end L102.end
  constraint coincident L6.end L103.start
  constraint coincident L98 L103.end
  constraint perpendicular L98 L103
  constraint coincident L19.start L104.start
  constraint coincident L99 L104.end
  constraint perpendicular L19 L104
  constraint coincident L99 L105.end
  constraint coincident L98 L105.end
  constraint coincident L65 L108.end
  constraint perpendicular L65 L108
  constraint perpendicular L38 L112
  constraint perpendicular L35 L113
  constraint coincident L38 L114.start
  constraint coincident L112 L114.start
  constraint coincident L112 L114.end
  constraint coincident L113 L114.end
  constraint coincident L113 L115.end
  constraint coincident L39 L115.end
  constraint perpendicular L114 L116
  constraint parallel L114 L118
  constraint coincident L118 A1.centre
  constraint coincident L116 A1.centre
  constraint perpendicular L8 L119
  constraint perpendicular L119 L120
  constraint perpendicular L119 L121
  constraint perpendicular L121 L122
  constraint coincident L119 L123.end
  constraint coincident L0 L123.end
  constraint coincident L120 L124.end
  constraint coincident L37 L124.end
  constraint coincident L122 A2.centre
  constraint coincident L121 A2.centre
  constraint perpendicular L8 L125
  constraint horizontal L126
  constraint perpendicular L6 L127
  constraint perpendicular L34 L128
  constraint coincident L125 L129.start
  constraint coincident L36 L129.start
  constraint coincident L126 L129.end
  constraint coincident L125 L129.end
  constraint coincident L2 L130.end
  constraint coincident L126 L130.end
  constraint coincident L128 A3.centre
  constraint coincident L127 A3.centre
  constraint parallel L3 L131
  constraint perpendicular L131 L132
  constraint horizontal L133
  constraint vertical L134
  constraint horizontal L135
  constraint vertical L136
  constraint coincident L131 L133.start
  constraint coincident L132 L133.start
  constraint perpendicular L135 L137
  constraint perpendicular L137 L138
  constraint coincident L138 A4.centre
  constraint coincident L137 A4.centre
  constraint midpoint L139 A5.centre
  measures "d104" distance of L0 L6
  measures "d105" distance of L1 L17
  measures "d106" distance of L5 L33
  measures "d107" distance of L4 L12
  measures "d108" distance of L2 L19
  measures "d116" distance of L30 L42
  measures "d117" distance of L43 L44
  measures "d118" distance of L39 L45
  measures "d119" distance of L32 L46
  measures "d120" distance of L28 L47
  measures "d121" distance of L12 L48
  measures "d122" distance of L29 L49
  measures "d123" distance of L10 L50
  measures "d124" distance of L13 L51
  measures "d125" distance of L31 L52
  measures "d127" distance of L53 L56
  measures "d128" distance of L30 L59
  measures "d129" diameter of A0
  measures "d130" distance of L39 A0.centre
  measures "d131" distance of L14 L81
  measures "d132" distance of L16 L82
  measures "d133" distance of L26 L83
  measures "d134" distance of L15 L84
  measures "d136" distance of L93 L96
  measures "d137" distance of L91 L95
  measures "d138" distance of L40 L99
  measures "d139" distance of L41 L98
  measures "d140" distance of L38 L97
  measures "d187" distance of L37 L113
  measures "d188" distance of L35 L112
  measures "d189" diameter of A1
  measures "d190" distance of L36 L120
  measures "d191" distance of L37 L119
  measures "d192" distance of L37 L122
  measures "d193" distance of L36 L121
  measures "d194" diameter of A2
  measures "d195" distance of L34 L125
  measures "d196" distance of L0 L126
  measures "d197" distance of L34 L127
  measures "d198" distance of L36 L128
  measures "d199" diameter of A3
  measures "d200" distance of L65 L131
  measures "d201" distance of L60 L132
  measures "d202" diameter of A4
  measures "d221" diameter of A5
extrude "Extrude1''''" add sketch "Box side view" along normal mid plane 40 separate body contours L34 L36 L40 L104 L105 L106 L129 L130 A3 | L34 L40 L79 L130 | L36 L41 L103 L106 L123 L129 | L36 L37 L38 L41 L100 L101 L102 L123 L124 A2 | L34 L40 L74 L80 | L106 A3 | L40 L68 L76 L77 | L34 L35 L37 L38 L39 L71 L72 L73 L75 A1 L124 | L41 A2 | L40 L67 L68 L76 | L63 L64 L68 L69 L70 L76 | L65 L66 L78 L108 | L105 A3 | L38 A2 | L60 L62 L63 L64 L65 L66 L108 L134 | L38 A1 | L39 A1 | L39 L56 L57 L58 | L53 L54 L55 L60 | L85 L86 L87 L88 L89 L90 L91 L92 L93 L94 L95 L96 makes body 5 at (6.6667, 8.95, -7.7) makes body 6 at (-6.6667, -21, 31.5733) makes body 7 at (6.6667, 7.9, 24.3833) in component "Box"
extrude "Extrude2''''" add sketch "Box side view" along normal blind 17 and the other way blind -20 contours L40 L41 L129 L130 A3 | L38 L39 L40 L41 L55 L58 L65 L78 L107 L111 L114 L115 L123 L124 L129 L130 L133 L135 L136 | L40 L66 L69 L77 L78 L107 L108 | L38 L41 L123 L124 A2 | L40 L68 L76 L77 | L40 L41 A3 | L38 L41 A2 | L40 L67 L68 L76 | L39 L40 L62 L67 L68 L76 L109 | L63 L64 L68 L69 L70 L76 | L65 L66 L78 L108 | L40 L41 A3 | L38 L41 A2 | L64 L66 L70 L108 | L60 L62 L63 L64 L65 L66 L108 L134 | L38 L39 L114 L115 A1 | L38 L39 A1 | L39 L54 L57 L60 L109 L110 | L65 L133 L134 L135 L136 | L38 L39 A1 | L39 L56 L57 L58 | L53 L54 L55 L60 | L53 L56 L110 L111 | L85 L86 L87 L88 L89 L90 L91 L92 L93 L94 L95 L96 | A4 | A5 bodies 5 6 7 in component "Box"
extrude "Extrude3'''" add sketch "Box side view" along normal blind 20 and the other way blind -17 contours L41 L103 L106 L129 | L41 L106 L129 A3 | L40 L104 L105 A3 | L41 L106 A3 | L40 L105 A3 | L40 L41 L105 L106 A3 | L38 L100 L101 L102 | L39 L71 L72 L73 bodies 5 in component "Box"
sketch "Box bottom view" plane through (0, 0, 0) normal (0, 0, 1) x (1, 0, 0)
  circle A0 centre (-11.3, -23.15) radius 1.6
  circle A1 centre (-11.3, 23.15) radius 1.6
  circle A2 centre (11.3, -23.15) radius 1.6
  circle A3 centre (11.3, 23.15) radius 1.6
  line L0 (4.4, -25.95) -> (4.4, -20.65)
  line L1 (4.4, -20.65) -> (-4.4, -20.65)
  line L2 (-4.4, -20.65) -> (-4.4, -25.95)
  line L3 (-4.4, -25.95) -> (-14.1, -25.95)
  line L4 (-14.1, -25.95) -> (-14.1, 25.95)
  line L5 (-14.1, 25.95) -> (14.1, 25.95)
  line L6 (14.1, 25.95) -> (14.1, -25.95)
  line L7 (14.1, -25.95) -> (4.4, -25.95)
  line L8 (8.9, -24.25) -> (8.9, -20.35)
  line L9 (8.9, -20.35) -> (6.3, -20.35)
  line L10 (6.3, -20.35) -> (6.3, -24.25)
  line L11 (6.3, -24.25) -> (8.9, -24.25)
  line L12 (-6.3, -24.25) -> (-6.3, -20.35)
  line L13 (-6.3, -20.35) -> (-8.9, -20.35)
  line L14 (-8.9, -20.35) -> (-8.9, -24.25)
  line L15 (-8.9, -24.25) -> (-6.3, -24.25)
  line L16 (2.9, -3.05) -> (2.9, -2.05)
  line L17 (2.9, -2.05) -> (0.9, -2.05)
  line L18 (0.9, -2.05) -> (0.9, -3.05)
  line L19 (0.9, -3.05) -> (2.9, -3.05)
  line L20 (-3.8, -3.05) -> (-3.8, -2.05)
  line L21 (-3.8, -2.05) -> (-5.8, -2.05)
  line L22 (-5.8, -2.05) -> (-5.8, -3.05)
  line L23 (-5.8, -3.05) -> (-3.8, -3.05)
  circle A4 centre (7.6, -22.3) radius 0.8
  circle A5 centre (-7.6, -22.3) radius 0.8
  line L24 (0.4, -3.55) -> (3.4, -3.55)
  line L25 (3.4, -3.55) -> (3.4, -1.55)
  line L26 (3.4, -1.55) -> (0.4, -1.55)
  line L27 (0.4, -1.55) -> (0.4, -3.55)
  line L28 (-3.3, -1.55) -> (-6.3, -1.55)
  line L29 (-6.3, -1.55) -> (-6.3, -3.55)
  line L30 (-6.3, -3.55) -> (-3.3, -3.55)
  line L31 (-3.3, -3.55) -> (-3.3, -1.55)
  circle A6 centre (7.6, -22.3) radius 1.3
  circle A7 centre (-7.6, -22.3) radius 1.3
  circle A8 centre (11.3, -23.15) radius 1.4
  circle A9 centre (11.3, 23.15) radius 1.4
  circle A10 centre (-11.3, 23.15) radius 1.4
  circle A11 centre (-11.3, -23.15) radius 1.4
  line L32 (15.3127, 20.15) -> (-15.4854, 20.15) construction
  line L33 (16.1574, -20.15) -> (-16.1352, -20.15) construction
  line L34 (15.5345, -26.15) -> (-16.1083, -26.15) construction
  line L35 (14.3, -28.0632) -> (14.3, -17.7322) construction
  line L36 (-14.3, -29.1678) -> (-14.3, -17.7322) construction
  line L37 (-9.4, -28.3231) -> (-9.4, -18.6418) construction
  line L38 (9.4, -28.3231) -> (9.4, -17.5373) construction
  line L39 (14.6898, 26.15) -> (-16.5631, 26.15) construction
  line L40 (-14.3, 18.5888) -> (-14.3, 28.7899) construction
  line L41 (14.3, 19.2386) -> (14.3, 28.7899) construction
  line L42 (9.4, 29.8295) -> (9.4, 19.2386) construction
  line L43 (-9.4, 29.8295) -> (-9.4, 19.2386) construction
  line L44 (14.3, -20.15) -> (9.4, -20.15)
  line L45 (9.4, -20.15) -> (9.4, -26.15)
  line L46 (9.4, -26.15) -> (14.3, -26.15)
  line L47 (14.3, -26.15) -> (14.3, -20.15)
  line L48 (-9.4, -20.15) -> (-14.3, -20.15)
  line L49 (-14.3, -20.15) -> (-14.3, -26.15)
  line L50 (-14.3, -26.15) -> (-9.4, -26.15)
  line L51 (-9.4, -26.15) -> (-9.4, -20.15)
  line L52 (9.4, 20.15) -> (14.3, 20.15)
  line L53 (14.3, 20.15) -> (14.3, 26.15)
  line L54 (14.3, 26.15) -> (9.4, 26.15)
  line L55 (9.4, 26.15) -> (9.4, 20.15)
  line L56 (-9.4, 20.15) -> (-14.3, 20.15)
  line L57 (-14.3, 20.15) -> (-14.3, 26.15)
  line L58 (-14.3, 26.15) -> (-9.4, 26.15)
  line L59 (-9.4, 26.15) -> (-9.4, 20.15)
  dimension "d145" = 0.5
  dimension "d146" = 0.5
  dimension "d147" = 0.5
  dimension "d148" = 0.5
  dimension "d149" = -0.2
  dimension "d150" = -0.2
  dimension "d151" = -0.2
  dimension "d152" = -0.2
  dimension "d153" = 3
  dimension "d154" = 3
  dimension "d155" = 3
  dimension "d156" = 0.5
  dimension "d157" = 0.5
  dimension "d158" = 3
  dimension "d159" = 3
  dimension "d160" = 3
  constraint perpendicular L4 L32
  constraint perpendicular L4 L33
  constraint perpendicular L4 L34
  constraint perpendicular L34 L35
  constraint perpendicular L34 L36
  constraint perpendicular L33 L37
  constraint perpendicular L33 L38
  constraint perpendicular L4 L39
  constraint perpendicular L39 L40
  constraint perpendicular L39 L41
  constraint perpendicular L32 L42
  constraint perpendicular L32 L43
  constraint collinear L38 L42
  constraint collinear L37 L43
  constraint collinear L36 L40
  constraint collinear L35 L41
  constraint horizontal L44
  constraint vertical L45
  constraint horizontal L46
  constraint vertical L47
  constraint coincident L34 L45.end
  constraint coincident L38 L45.end
  constraint coincident L33 L44.start
  constraint coincident L35 L44.start
  constraint horizontal L48
  constraint vertical L49
  constraint horizontal L50
  constraint vertical L51
  constraint coincident L34 L49.end
  constraint coincident L36 L49.end
  constraint coincident L37 L48.start
  constraint coincident L33 L48.start
  constraint horizontal L52
  constraint vertical L53
  constraint horizontal L54
  constraint vertical L55
  constraint coincident L41 L53.end
  constraint coincident L39 L53.end
  constraint coincident L32 L52.start
  constraint coincident L42 L52.start
  constraint horizontal L56
  constraint vertical L57
  constraint horizontal L58
  constraint vertical L59
  constraint coincident L40 L57.end
  constraint coincident L39 L57.end
  constraint coincident L32 L56.start
  constraint coincident L43 L56.start
  measures "d153" distance of A3.centre L41
  measures "d154" distance of A3.centre L39
  measures "d155" distance of A1.centre L40
  measures "d156" distance of L8 L38
  measures "d157" distance of L14 L37
  measures "d158" distance of A3.centre L32
  measures "d159" distance of A0.centre L48
  measures "d160" distance of A0.centre L50
extrude "Extrude4''" cut sketch "Box bottom view" against normal blind 10 contours A6 | A7 | L16 L17 L18 L19 | L20 L21 L22 L23 | A4 | A5 | L24 L25 L26 L27 | L28 L29 L30 L31 bodies 5 in component "Box"
extrude "Extrude5''" add sketch "Box bottom view" along normal blind -7 and the other way blind 1 contours A0 | A1 | A2 | A3 | L6 L7 L44 L45 | L3 L4 L48 L51 | L5 L6 L52 L55 | L4 L5 L56 L59 | A8 | A9 | A10 | A11 bodies 5 in component "Box"
extrude "Extrude6'" add sketch "Box bottom view" along normal blind 1 and the other way blind 1 contours A8 | A9 | A10 | A11 bodies 5 in component "Box"
fillet "Fillet1" radius 1 4 edges at (-12.6053, -23.6563, 1) (9.9947, -23.6563, 1) (-12.6053, 22.6437, 1) (9.9947, 22.6437, 1) on bodies 5 in component "Box"
fillet "Fillet2" radius 3 12 edges at (-14.1, 23.05, -4.7) (-14.1, -23.3, -4.9) (9.4, -23.3, -4.9) (9.4, 23.05, -4.7) (-9.4, 23.05, -4.7) (14.1, 23.05, -4.7) (-9.4, -23.3, -4.9) (14.1, -23.3, -4.9) (11.75, 20.15, -4.7) (-11.75, 20.15, -4.7) (11.75, -20.15, -4.7) (-11.75, -20.15, -4.7) on bodies 5 in component "Box"
extrude "Extrude7" add sketch "Box side view" along normal blind 20 and the other way blind -9 contours L34 L40 L79 L80 | L40 L66 L69 L77 L78 L107 L108 | L64 L66 L70 L108 bodies 5 in component "Box"
extrude "Extrude8" add sketch "Box side view" along normal blind 20 and the other way blind -15 contours L34 L40 L74 L75 bodies 5 in component "Box"
extrude "Extrude9" add sketch "Box side view" along normal blind 17.5 and the other way blind -2.5 contours L39 L54 L57 L60 L109 L110 | L53 L56 L110 L111 bodies 5 in component "Box"
extrude "Extrude10" add sketch "Box side view" along normal mid plane 40 contours L38 L39 L114 L115 A1 | L65 L133 L134 L135 L136 bodies 5 in component "Box"
extrude "Extrude11" add sketch "Box side view" along normal blind -15 and the other way blind 20 contours L34 L36 L40 L104 L105 L106 L129 L130 A3 | L40 L41 L129 L130 A3 | L36 L37 L38 L41 L100 L101 L102 L123 L124 A2 | L41 L106 L129 A3 | L40 L104 L105 A3 | L38 L41 L123 L124 A2 | L40 L41 L105 L106 A3 | L38 L100 L101 L102 bodies 5 in component "Box"
fillet "Fillet3" radius 0.75 2 edges at (-15.9658, 20.9615, -4.4773) (-18.55, 20.9607, -4.7) on bodies 5 in component "Box"
fillet "Fillet4" radius 1.5 1 edges at (-17.5, 25.95, 0.3) on bodies 5 in component "Box"
fillet "Fillet5" radius 2.5 1 edges at (-17.5, -28.05, 0.3) on bodies 5 in component "Box"
fillet "Fillet6" radius 0.75 2 edges at (-18.55, -23.05, -4.9) (-15.9658, -23.05, -4.6773) on bodies 5 in component "Box"
fillet "Fillet7" radius 3 5 edges at (-1.5, 20.95, 40.05) (-1.5, -13, 31.95) (-17.5, 20.9786, 0.3) (-1.5, -13, 39.95) (-17.5, -23.05, 0.3) on bodies 5 in component "Box"
fillet "Fillet8" radius 1.5 6 edges at (-1.5, 7.9, 29.15) (-1.5, 22.1, 29.15) (-1.5, 7.9, 14.85) (-1.5, 22.1, 14.85) (-1.5, 19.1, 14.85) (-1.5, 10.9, 14.85) on bodies 5 in component "Box"
extrude "Extrude12" cut sketch "Box side view" along normal blind 20 and the other way blind -17 contours A5 bodies 5 in component "Box"
component "Light sensor" placed x (1, 0, 0) y (0, 0, 1) z (0, -1, 0) at (0, -23, 43)
component "ESP32 Wroom-32" placed x (1, 0, 0) y (0, -1, 0) z (0, 0, -1) at (0, 0, 0)
component "Screw terminal" placed x (0, 1, 0) y (0, 0, -1) z (-1, 0, 0) at (0, 15, 22)
component "DHT22" placed x (1, 0, 0) y (0, 0, 1) z (0, -1, 0) at (0, -23, 20)
component "Box" placed x (1, 0, 0) y (0, 1, 0) z (0, 0, 1) at (0, 0, 0)
equation "d3 = ( 20 / 2 ) * 1 mm + 5 mm"
equation "d16 = ( 7.7 / 2 ) * 1 mm + 0.25 mm"
equation "d18 = ( -7.7 / 2 ) * 1 mm + 0.25 mm"
equation "d37 = ( 3.2 / 2 ) * 1 mm + 1.2 mm"
equation "d38 = ( 3.2 / 2 ) * 1 mm + 1.2 mm"
equation "d60 = 1.5 mm + 3.2 mm"
equation "d64 = 1.5 mm + 2 mm"
equation "d68 = 1.5 mm + 2.2 mm + 0.5 mm"
equation "d72 = 1.5 mm + 0.5 mm"
equation "d92 = ( 7.7 / 2 ) * 1 mm + 0.3 mm"
equation "d94 = ( -7.7 / 2 ) * 1 mm"
